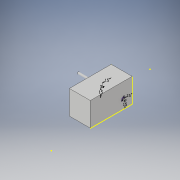
# Autodesk Inventor part: Motor_links
Saved by Autodesk Inventor 2019.5 (Build 235369000, 369)
## iProperties
Created: 2021-09-30
Part Number: Motor_links
Material: Generisch
Document SubType Name: Modeling
Designer: mritt
Density: 1 g/cm^3
Appearance: Vorgabe
Author: mritt
Autodesk Inventor part; units mm, degrees
ref_plane "YZ Plane" through (0, 0, 0) normal (1, 0, 0) x (0, 1, 0)
ref_plane "XZ Plane" through (0, 0, 0) normal (0, 1, 0) x (-1, 0, 0)
ref_plane "XY Plane" through (0, 0, 0) normal (0, 0, 1) x (1, 0, 0)
sketch "Skizze1" plane through (0, 0, 0) normal (0, 1, 0) x (-1, 0, 0)
  line L0 (52.027, -65.0338) -> (17.027, -65.0338)
  line L1 (17.027, -65.0338) -> (17.027, -135.0338)
  line L2 (17.027, -135.0338) -> (52.027, -135.0338)
  line L3 (52.027, -135.0338) -> (52.027, -65.0338)
  point P0 (0, 0)
  dimension "d0" = 70
  dimension "d1" = 35
  constraints: 8 end point, 2 parallel, 1 horizontal, 1 perpendicular
  measures "d0" distance of L2.end L0.start
  measures "d1" distance of L1.end L2.end
extrude "Extrusion1" add sketch "Skizze1" along normal blind 40
sketch "Skizze2" plane through (-17.027, 0, -65.0338) normal (1, 0, 0) x (0, 0, -1)
  circle A0 centre (55, 15) radius 1.5
  circle A1 centre (55, 15) radius 2.5
  line L0 (0, 0) -> (70, 0) projected
  line L1 (70, 0) -> (70, 40) projected
  point P0 (-65.0338, 0)
  dimension "d4" = 3
  dimension "d5" = 5
  dimension "d6" = 15
  dimension "d7" = 15
  constraints: 2 centre point, 1 coincident
  measures "d4" diameter of A0
  measures "d5" diameter of A1
  measures "d6" distance from line of A0.centre L0
  measures "d7" distance from line of A0.centre L1
extrude "Extrusion2" add sketch "Skizze2" along normal blind 4 contours A0
extrude "Extrusion3" add sketch "Skizze2" along normal blind 1
sketch "Skizze3" plane through (-52.027, 0, -135.0338) normal (-1, 0, 0) x (0, 0, 1)
  circle A0 centre (15, 15) radius 1.5
  circle A1 centre (15, 15) radius 2.5
  line L0 (0, 0) -> (0, 40) projected
  line L1 (0, 0) -> (70, 0) projected
  point P0 (-65.0338, 0)
  dimension "d12" = 3
  dimension "d13" = 5
  dimension "d16" = 15
  dimension "d17" = 15
  constraints: 2 centre point, 1 coincident
  measures "d12" diameter of A0
  measures "d13" diameter of A1
  measures "d16" distance from line of A0.centre L0
  measures "d17" distance from line of A0.centre L1
extrude "Extrusion4" add sketch "Skizze3" along normal blind 40 contours A0
extrude "Extrusion5" add sketch "Skizze3" along normal blind 10
